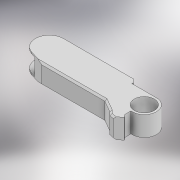
# Autodesk Inventor part: Lower Leg
Saved by Autodesk Inventor 2022 (Build 260153000, 153)
## iProperties
Created: 2022-02-26
Part Number: Lower Leg
Material: Generic
Document SubType Name: Modeling
Designer: joshw
Density: 1 g/cm^3
Appearance: Default
Author: joshw
Autodesk Inventor part; units mm, degrees
ref_plane "YZ Plane" through (0, 0, 0) normal (1, 0, 0) x (0, 1, 0)
ref_plane "XZ Plane" through (0, 0, 0) normal (0, 1, 0) x (-1, 0, 0)
sketch "Sketch1" plane through (0, 0, 0) normal (0, 1, 0) x (-1, 0, 0)
  circle A0 centre (18.719305, 0.91995) radius 3.625
  line L0 (19.118903, 4.522858) -> (19.118903, 6.41995)
  line L1 (19.118903, 6.41995) -> (18.491054, 7.168191)
  line L2 (18.491054, 7.168191) -> (20.291054, 8.668191)
  line L3 (20.291054, 8.668191) -> (21.541054, 8.418191)
  line L4 (21.541054, 8.418191) -> (22.541054, 7.418191)
  line L5 (22.541054, 7.418191) -> (26.041054, 5.418191)
  line L6 (26.041054, -4.16305) -> (26.041054, 5.418191)
  line L7 (26.041054, 5.418191) -> (45.041054, 5.418191)
  line L8 (45.041054, 5.418191) -> (49.279808, 4.102266)
  line L9 (18.849216, -2.702721) -> (26.041054, -2.702721)
  circle A1 centre (48.026329, 0.064657) radius 4.227707
  line L10 (48.026329, -4.16305) -> (26.041054, -4.16305)
  circle A2 centre (18.719305, 0.91995) radius 3
  point P0 (0, 0)
  dimension "d0" = 7.25
  dimension "d1" = 5.5
  dimension "d2" = 140
  dimension "d3" = 1.5
  dimension "d4" = 1.8
  dimension "d5" = 1.25
  dimension "d6" = 0.25
  dimension "d7" = 1
  dimension "d8" = 1
  dimension "d9" = 3.5
  dimension "d10" = 2
  dimension "d11" = 19
  dimension "d12" = 6
  dimension "d15" = 5.083
  constraints: 23 end point, 4 point on circle, 3 centre point, 2 parallel, 2 tangent, 1 coincident, 1 horizontal, 1 point on line, 1 vertical
  measures "d0" diameter of A0
  measures "d1" vertical distance of L0.end A0.centre
  measures "d2" angle of L0 L1
  measures "d3" vertical distance of L1.end L2.end
  measures "d4" horizontal distance of L1.end L2.end
  measures "d5" horizontal distance of L2.end L3.end
  measures "d6" vertical distance of L2.end L3.end
  measures "d7" horizontal distance of L3.end L4.end
  measures "d8" horizontal distance of L3.end L4.end
  measures "d9" horizontal distance of L4.end L5.end
  measures "d10" vertical distance of L4.end L5.end
  measures "d11" distance of L5.end L7.end
  measures "d12" diameter of A2
  measures "d15" distance from line of L10 A0.centre
extrude "Extrusion1" add sketch "Sketch1" along normal mid plane 5.95
ref_plane "Work Plane1" through (-52.254036, 0, 0.064657) normal (1, 0, 0) x (0, 0, -1)
sketch "Sketch2" plane through (-52.254036, 0, 0.064657) normal (1, 0, 0) x (0, 0, -1)
  point P0 (0.064657, 0)
sketch "Sketch3" plane through (-52.254036, 0, 0.064657) normal (1, 0, 0) x (0, 0, -1)
  line L0 (-4.03761, -2.975) -> (4.227707, -2.975) construction
  line L1 (4.227707, 2.975) -> (-4.03761, 2.975) construction
  line L2 (-4.03761, -2.975) -> (-4.03761, 2.975) construction
  line L3 (2.767378, 2.975) -> (4.227707, 2.975) construction
  line L4 (-4.03761, -2.975) -> (4.227707, 2.975) construction
  line L5 (4.227707, -2.975) -> (4.227707, 2.975) construction
  line L6 (4.227707, -2.975) -> (0.095048, 0) construction
  line L7 (-3.654952, -2.5) -> (3.845048, -2.5)
  line L8 (3.845048, -2.5) -> (3.845048, 2.5)
  line L9 (3.845048, 2.5) -> (-3.654952, 2.5)
  line L10 (-3.654952, 2.5) -> (-3.654952, -2.5)
  line L11 (-3.654952, -2.5) -> (3.845048, 2.5) construction
  line L12 (3.845048, -2.5) -> (-3.654952, 2.5) construction
  point P0 (0.064657, 0)
  dimension "d16" = 7.5
  dimension "d17" = 5
  constraints: 16 end point, 3 midpoint, 2 parallel, 1 horizontal, 1 perpendicular
  measures "d16" distance of L9.end L8.end
  measures "d17" distance of L8.end L7.end
extrude "Extrusion2" cut sketch "Sketch3" along normal blind 8.25
sketch "Sketch4" plane through (-50.151142, -2.5, 3.719608) normal (0, 1, 0) x (1, 0, 0)
  arc A0 (2.124813, 7.882658) -> (0.871334, -0.382658) centre (2.124813, 3.654952) ccw
  circle A1 centre (2.124813, 3.654952) radius 2.55
  point P0 (50.151142, 3.719608)
  dimension "d20" = 5.1
  constraints: 1 centre point, 1 coincident
  measures "d20" diameter of A1
extrude "Extrusion3" add sketch "Sketch4" along normal up to surface (5 mm away)
sketch "Sketch5" plane through (-49.783914, -2.5, -3.780392) normal (0, 0, 1) x (1, 0, 0)
  line L0 (0, 0) -> (0, 5) projected
  line L1 (0, 0) -> (3.5, 0)
  line L2 (3.5, 0) -> (3.5, 5)
  line L3 (0, 5) -> (3.5, 5)
  point P0 (49.783914, 2.5)
  point P1 (3.5, 0.293722)
  dimension "d23" = 3.5
  constraints: 6 end point, 1 point on line
  measures "d23" distance from line of point (3.5, 0.294) L0
extrude "Extrusion4" cut sketch "Sketch5" against normal blind 4.25
sketch "Sketch6" plane through (-44.004036, 2.5, 3.719608) normal (0, 0, -1) x (-1, 0, 0)
  line L0 (6.147107, 0) -> (0, 0)
  line L1 (6.147107, 0) -> (4.147107, 0)
  line L2 (4.147107, 0) -> (4.147107, -5)
  line L3 (4.147107, -5) -> (6.147107, -5)
  line L4 (6.147107, -5) -> (6.147107, 0)
  line L5 (6.147107, -5) -> (0, -5)
  point P0 (-44.004036, -2.5)
  point P1 (4.147107, 0)
  dimension "d26" = 2
  constraints: 8 end point, 2 parallel, 1 collinear, 1 horizontal, 1 perpendicular
  measures "d26" distance of L3.end L2.end
extrude "Extrusion5" cut sketch "Sketch6" against normal blind 4.25
fillet "Fillet1" radius 0.3665 2 edges at (-48.1511, 0, 4.4527) (-48.1511, 0, 3.7196)
chamfer "Chamfer1" distance 0.5 angle 45 8 edges at (-35.5411, -2.975, 5.4182) (-35.5411, 2.975, 5.4182) (-24.2911, 2.975, 6.4182) (-24.2911, -2.975, 6.4182) (-22.0411, -2.975, 7.9182) (-22.0411, 2.975, 7.9182) (-20.9161, 2.975, 8.5432) (-20.9161, -2.975, 8.5432)
chamfer "Chamfer2" distance 1 angle 45 1 edges at (-26.0411, 0, -4.1631)
body "Solid1"
